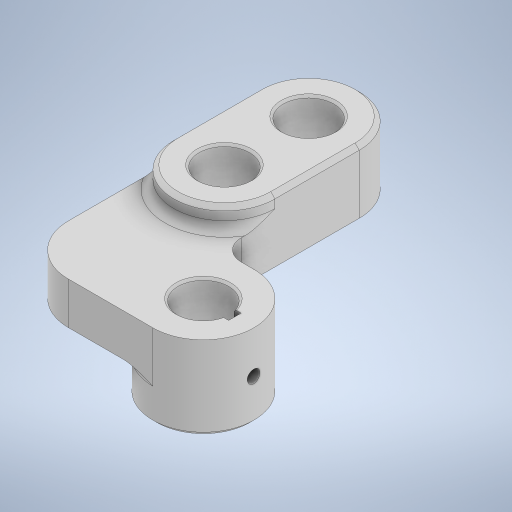
# Autodesk Inventor part: Week13_Homework01
Saved by Autodesk Inventor 2023 (Build 270158000, 158)
## iProperties
Created: 2023-05-22
Part Number: Week13_Homework01
Material: 一般
Document SubType Name: Modeling
Designer: m8317
Density: 1 g/cm^3
Appearance: 預設
Author: m8317
Autodesk Inventor part; units mm, degrees
ref_plane "YZ Plane" through (0, 0, 0) normal (1, 0, 0) x (0, 1, 0)
ref_plane "XZ Plane" through (0, 0, 0) normal (0, 1, 0) x (-1, 0, 0)
ref_plane "XY Plane" through (0, 0, 0) normal (0, 0, 1) x (1, 0, 0)
sketch "草圖1" plane through (0, 0, 0) normal (0, 1, 0) x (-1, 0, 0)
  line L0 (-12, 18.4299) -> (-12, -9.5701)
  line L1 (0, -21.5701) -> (0, -21.5701)
  line L2 (12, -9.5701) -> (12, 35.4299)
  circle A0 centre (0, -9.5701) radius 6
  circle A1 centre (0, 10.4299) radius 6
  line L3 (0, 47.4299) -> (-20, 47.4299)
  line L4 (-32, 35.4299) -> (-32, 35.4299)
  line L5 (-20, 23.4299) -> (-17, 23.4299)
  arc A2 (-25.8095, 33.9299) -> (-25.8095, 36.9299) centre (-20, 35.4299) ccw
  arc A3 (12, 35.4299) -> (0, 47.4299) centre (0, 35.4299) ccw
  arc A4 (-20, 47.4299) -> (-32, 35.4299) centre (-20, 35.4299) ccw
  arc A5 (-32, 35.4299) -> (-20, 23.4299) centre (-20, 35.4299) ccw
  arc A6 (-12, -9.5701) -> (0, -21.5701) centre (0, -9.5701) ccw
  arc A7 (0, -21.5701) -> (12, -9.5701) centre (0, -9.5701) ccw
  arc A8 (-12, 18.4299) -> (-17, 23.4299) centre (-17, 18.4299) ccw
  arc A9 (12, 10.4299) -> (-12, 10.4299) centre (0, 10.4299) ccw
  circle A10 centre (-20, 35.4299) radius 12
  line L6 (-27.5, 36.9299) -> (-27.5, 33.9299)
  line L7 (12, 35.4299) -> (-32, 35.4299) construction
  line L8 (0, -21.5701) -> (0, 47.4299) construction
  line L9 (-25.8095, 36.9299) -> (-27.5, 36.9299)
  line L10 (-27.5, 33.9299) -> (-25.8095, 33.9299)
  line L11 (-25.8095, 36.9299) -> (-25.8095, 33.9299) construction
  point P0 (0, 0)
  point P1 (0, -21.5701)
  point P2 (-20, 23.4299)
  point P3 (-25.8095, 35.4299)
  dimension "d0" = 24
  dimension "d1" = 12
  dimension "d2" = 12
  dimension "d3" = 20
  dimension "d4" = 24
  dimension "d5" = 12
  dimension "d6" = 45
  dimension "d7" = 20
  dimension "d8" = 32
  dimension "d9" = 12
  dimension "d10" = 12
  dimension "d11" = 12
  dimension "d12" = 5
  dimension "d22" = 3
  dimension "d23" = 7.5
  constraints: 24 end point, 16 point on circle, 13 tangent, 10 centre point, 5 point on line, 4 coincident, 4 equal radius, 4 perpendicular, 2 horizontal, 2 parallel, 1 midpoint, 1 vertical, 3 other
  measures "d0" distance between parallel lines of L0 L2
  measures "d1" diameter of A0
  measures "d2" diameter of A1
  measures "d3" distance of A0.centre A1.centre
  measures "d4" distance between parallel lines of L5 L3
  measures "d5" diameter of A2
  measures "d6" vertical distance of A0.centre A2.centre
  measures "d7" horizontal distance of A2.centre A1.centre
  measures "d8" distance from line of A2.centre L2
  measures "d9" distance from line of L1 A0.centre
  measures "d10" distance from line of L4 A2.centre
  measures "d11" radius of A3
  measures "d12" radius of A8
  measures "d22" distance of L6.start L6.end
  measures "d23" distance from line of A2.centre L6
extrude "擠出1" add sketch "草圖1" along normal blind 10
extrude "擠出2" add sketch "草圖1" along normal blind 5 from surface at 10 contours A9 L2 A7 A6 L0
extrude "擠出3" add sketch "草圖1" against normal blind 10 contours A5 A4 A10
chamfer "倒角1" distance 1 angle 45 5 edges at (0, 15, -21.5701) (12, 15, 0.4299) (0, 15, 22.4299) (-12, 15, 0.4299) (20, -10, 23.4299)
fillet "圓角1" radius 2 1 edges at (0, 10, 22.4299)
fillet "圓角2" radius 2 1 edges at (8, 0, 35.4299)
chamfer "倒角2" distance 0.5 angle 45 6 edges at (6, 15, 10.4299) (6, 15, -9.5701) (14, 10, 35.4299) (14, -10, 35.4299) (6, 0, 10.4299) (6, 0, -9.5701)
ref_plane "工作平面1" through (32, 0, 35.4299) normal (-1, 0, 0) x (0, 0, 1)
sketch "草圖2" plane through (32, 0, 35.4299) normal (-1, 0, 0) x (0, 0, 1)
  line L0 (1.5, -10) -> (-1.5, -10) construction
  line L1 (12, 10) -> (0, 10) construction
  line L2 (0, -10) -> (0, 10) construction
  line L3 (0, 0) -> (0, 10) construction
  circle A0 centre (0, 0) radius 1.5
  point P0 (-35.4299, 0)
  dimension "d29" = 3
  constraints: 2 end point, 1 centre point, 1 midpoint, 1 vertical
  measures "d29" diameter of A0
hole "孔1" at (32, 0, 35.4299) direction (-1, 0, 0) diameter 3 depth 5 tip angle 118 clearance for "Countersunk Flat Head Screw ISO 2009/7046" size "M3" standard "ISO"
